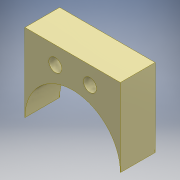
# Autodesk Inventor part: CubreRodamiento
Saved by Autodesk Inventor 2016 (Build 200138000, 138)
## iProperties
Created: 2019-03-18
Part Number: CubreRodamiento
Material: Nilón 6/6
Document SubType Name: Modeling
Designer: FIMCP
Mass: 1.73384 g
Surface Area: 12.7485 cm^2
Volume: 1.53437 cm^3
Density: 1.13 g/cm^3
Appearance: Nilón 6
Author: FIMCP
Autodesk Inventor part; units mm, degrees
ref_plane "YZ Plane" through (0, 0, 0) normal (1, 0, 0) x (0, 1, 0)
ref_plane "XZ Plane" through (0, 0, 0) normal (0, 1, 0) x (-1, 0, 0)
ref_plane "XY Plane" through (0, 0, 0) normal (0, 0, 1) x (1, 0, 0)
sketch "Boceto1" plane through (0, 0, 0) normal (0, 1, 0) x (-1, 0, 0)
  line L0 (0, 0) -> (-22, 0)
  line L1 (-22, 0) -> (-22, -18)
  line L2 (0, -18) -> (0, 0)
  arc A0 (0, -18) -> (-22, -18) centre (-11, -18) ccw
  circle A1 centre (-15, -4) radius 1.5
  circle A2 centre (-7, -4) radius 1.5
  dimension "d0" = 3
  dimension "d1" = 4
  dimension "d2" = 7
  dimension "d3" = 3
  dimension "d4" = 7
  dimension "d5" = 4
  constraints: 6 end point, 3 centre point, 2 point on circle, 1 horizontal, 1 parallel, 1 perpendicular
  measures "d0" diameter of A1
  measures "d1" distance from line of L0 A1.centre
  measures "d2" distance from line of L1 A1.centre
  measures "d3" diameter of A2
  measures "d4" distance from line of A2.centre L2
  measures "d5" distance from line of L0 A2.centre
extrude "Extrusión1" add sketch "Boceto1" along normal blind 8
